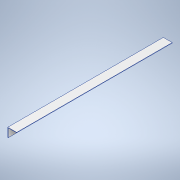
# Autodesk Inventor part: уголок 350
Saved by Autodesk Inventor 2022.4 (Build 264492010, 492A)
## iProperties
Created: 2023-02-20
Part Number: уголок 350
Material: Алюминий 6061
Document SubType Name: Modeling
Designer: artyo
Density: 2.7 g/cm^3
Appearance: Алюминий — плоский
Author: artyo
Autodesk Inventor part; units mm, degrees
ref_plane "YZ Plane" through (0, 0, 0) normal (1, 0, 0) x (0, 1, 0)
ref_plane "XZ Plane" through (0, 0, 0) normal (0, 1, 0) x (-1, 0, 0)
ref_plane "XY Plane" through (0, 0, 0) normal (0, 0, 1) x (1, 0, 0)
sketch "Эскиз2" plane through (0, 0, 0) normal (0, 0, 1) x (1, 0, 0)
  line L0 (0, 0) -> (0.5, 0)
  line L1 (0.5, 0) -> (-0.5, 0)
  line L2 (-0.5, 0) -> (-0.5, 20)
  line L3 (-0.5, 20) -> (19.5, 20)
  line L4 (19.5, 20) -> (19.5, 19)
  line L5 (19.5, 19) -> (0.5, 19)
  line L6 (0.5, 19) -> (0.5, 0)
  dimension "d0" = 0.5
  dimension "d1" = 1
  dimension "d2" = 20
  dimension "d3" = 20
  dimension "d4" = 1
  constraints: 14 end point, 3 perpendicular, 1 horizontal, 1 parallel, 1 point on line, 1 vertical
  measures "d0" distance of L0.start L0.end
  measures "d1" distance of L0.end L1.end
  measures "d2" distance of L1.end L2.end
  measures "d3" distance of L2.end L3.end
  measures "d4" distance of L3.end L4.end
extrude "Выдавливание1" add sketch "Эскиз2" along normal blind 350
